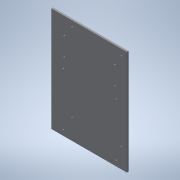
# Autodesk Inventor part: Akrilik
Saved by Autodesk Inventor 2020 (Build 240168000, 168)
## iProperties
Created: 2021-04-23
Part Number: Akrilik
Material: Generic
Document SubType Name: Modeling
Designer: scrip
Density: 1 g/cm^3
Appearance: Default
Author: scrip
Autodesk Inventor part; units mm, degrees
ref_plane "YZ Plane" through (0, 0, 0) normal (1, 0, 0) x (0, 1, 0)
ref_plane "XZ Plane" through (0, 0, 0) normal (0, 1, 0) x (-1, 0, 0)
ref_plane "XY Plane" through (0, 0, 0) normal (0, 0, 1) x (1, 0, 0)
sketch "Sketch1" plane through (0, 0, 0) normal (0, 0, 1) x (1, 0, 0)
  line L0 (-43.437, -19.7437) -> (55.293, -19.7437)
  line L1 (55.293, -19.7437) -> (55.293, -118.7837)
  circle A0 centre (6.169, -65.1647) radius 0.508
  circle A1 centre (-0.333, -65.1647) radius 0.508
  arc A2 (23.1745, -85.9924) -> (23.1745, -82.9951) centre (23.238, -84.4937) ccw
  arc A3 (23.1745, -82.9951) -> (23.1745, -85.9924) centre (23.111, -84.4937) ccw
  circle A4 centre (-11.179, -100.7497) radius 0.75
  circle A5 centre (28.445, -83.4777) radius 0.75
  circle A6 centre (36.573, -92.1137) radius 0.508
  circle A7 centre (-30.737, -64.3737) radius 0.4
  circle A8 centre (-25.657, -64.3737) radius 0.4
  circle A9 centre (-33.277, -89.3737) radius 0.4
  circle A10 centre (-28.197, -89.3737) radius 0.4
  circle A11 centre (-23.117, -89.3737) radius 0.4
  circle A12 centre (-12.957, -41.3137) radius 0.508
  circle A13 centre (-7.877, -41.3137) radius 0.508
  circle A14 centre (-12.957, -32.4237) radius 0.508
  circle A15 centre (-7.877, -32.4237) radius 0.508
  circle A16 centre (-25.657, -98.4637) radius 0.508
  circle A17 centre (-30.737, -98.4637) radius 0.508
  circle A18 centre (-29.467, -32.4237) radius 0.508
  circle A19 centre (-24.387, -32.4237) radius 0.508
  circle A20 centre (-14.227, -60.3637) radius 0.55
  circle A21 centre (-32.007, -71.7937) radius 0.508
  circle A22 centre (-26.927, -71.7937) radius 0.508
  circle A23 centre (-21.847, -71.7937) radius 0.508
  circle A24 centre (-14.227, -71.7937) radius 0.508
  circle A25 centre (-9.147, -71.7937) radius 0.508
  circle A26 centre (-4.067, -71.7937) radius 0.508
  circle A27 centre (-32.007, -23.5337) radius 0.508
  circle A28 centre (-26.927, -23.5337) radius 0.508
  circle A29 centre (-21.847, -23.5337) radius 0.508
  circle A30 centre (-16.767, -23.5337) radius 0.508
  circle A31 centre (-10.163, -23.5337) radius 0.508
  circle A32 centre (-5.083, -23.5337) radius 0.508
  circle A33 centre (-0.003, -23.5337) radius 0.508
  circle A34 centre (5.077, -23.5337) radius 0.508
  circle A35 centre (-39.627, -23.5337) radius 1.5
  circle A36 centre (51.813, -114.9737) radius 1.5
  circle A37 centre (-37.087, -38.7737) radius 1.6
  circle A38 centre (-7.877, -51.4737) radius 0.55
  circle A39 centre (-9.147, -60.3637) radius 0.55
  circle A40 centre (-7.877, -46.3937) radius 0.55
  circle A41 centre (13.713, -23.5337) radius 1.6
  circle A42 centre (-37.087, -66.7137) radius 1.6
  circle A43 centre (-39.627, -114.9737) radius 1.5
  circle A44 centre (51.813, -23.5337) radius 1.5
  circle A45 centre (2.537, -23.5337) radius 0.508
  circle A46 centre (-2.543, -23.5337) radius 0.508
  circle A47 centre (-7.623, -23.5337) radius 0.508
  circle A48 centre (-12.703, -23.5337) radius 0.508
  circle A49 centre (-19.307, -23.5337) radius 0.508
  circle A50 centre (-24.387, -23.5337) radius 0.508
  circle A51 centre (-29.467, -23.5337) radius 0.508
  circle A52 centre (-34.547, -23.5337) radius 0.508
  circle A53 centre (-6.607, -71.7937) radius 0.508
  circle A54 centre (-11.687, -71.7937) radius 0.508
  circle A55 centre (-16.767, -71.7937) radius 0.508
  circle A56 centre (-24.387, -71.7937) radius 0.508
  circle A57 centre (-29.467, -71.7937) radius 0.508
  circle A58 centre (-34.547, -71.7937) radius 0.508
  circle A59 centre (-21.847, -32.4237) radius 0.508
  circle A60 centre (-26.927, -32.4237) radius 0.508
  circle A61 centre (-33.277, -98.4637) radius 0.508
  circle A62 centre (-28.197, -98.4637) radius 0.508
  circle A63 centre (-5.337, -32.4237) radius 0.508
  circle A64 centre (-10.417, -32.4237) radius 0.508
  circle A65 centre (-5.337, -41.3137) radius 0.508
  circle A66 centre (-10.417, -41.3137) radius 0.508
  circle A67 centre (-20.577, -89.3737) radius 0.4
  circle A68 centre (-25.657, -89.3737) radius 0.4
  circle A69 centre (-30.737, -89.3737) radius 0.4
  circle A70 centre (-23.117, -64.3737) radius 0.4
  circle A71 centre (-28.197, -64.3737) radius 0.4
  circle A72 centre (36.573, -89.5737) radius 0.508
  circle A73 centre (36.573, -94.6537) radius 0.508
  circle A74 centre (28.445, -100.7497) radius 0.75
  circle A75 centre (-11.179, -83.4777) radius 0.75
  circle A76 centre (-6.607, -99.7337) radius 1.5
  circle A77 centre (-0.333, -60.6427) radius 0.508
  circle A78 centre (6.169, -60.6427) radius 0.508
  line L2 (55.293, -118.7837) -> (-43.437, -118.7837)
  line L3 (55.293, -19.7437) -> (55.293, -118.7837)
  line L4 (-43.437, -19.7437) -> (55.293, -19.7437)
  line L5 (-43.437, -118.7837) -> (-43.437, -19.7437)
  line L6 (-59.627, 55.0712) -> (-59.627, -124.9737)
  line L7 (-59.627, -124.9737) -> (70.373, -124.9737)
  line L8 (70.373, -124.9737) -> (70.373, 55.0712)
  line L9 (70.373, 55.0712) -> (-59.627, 55.0712)
  arc A79 (-37.9994, -7.7176) -> (-37.9994, -3.2176) centre (-37.9994, -5.4676) ccw
  arc A80 (-37.9994, 23.973) -> (-37.9994, 28.473) centre (-37.9994, 26.223) ccw
  arc A81 (49.0006, -3.2176) -> (49.0006, -7.7176) centre (49.0006, -5.4676) ccw
  arc A82 (49.0006, 28.473) -> (49.0006, 23.973) centre (49.0006, 26.223) ccw
  circle A83 centre (-39.627, -23.5337) radius 1.5
  circle A84 centre (-39.627, -114.9737) radius 1.5
  circle A85 centre (51.813, -114.9737) radius 1.5
  circle A86 centre (51.813, -23.5337) radius 1.5
  circle A87 centre (49.0006, -5.4676) radius 1.5
  circle A88 centre (49.0006, 26.223) radius 1.5
  circle A89 centre (-37.9994, 26.223) radius 1.1903
  circle A90 centre (-37.9994, -5.4676) radius 1.5
  point P0 (0, 0)
  point P1 (-30.337, -14.7437)
  point P2 (19.4617, -123.7837)
  point P3 (60.293, -53.7773)
  point P4 (-48.437, -58.5398)
extrude "Extrusion1" add sketch "Sketch1" along normal blind 3 contours L0 L1 L2 L5 | A0 | A1 | A3 A2 | A4 | A5 | A6 | A7 | A8 | A9 | A10 | A11 | A12 | A13 | A14 | A15 | A16 | A17 | A18 | A19 | A20 | A21 | A22 | A23 | A24 | A25 | A26 | A27 | A28 | A29 | A30 | A31 | A32 | A33 | A34 | A35 | A36 | A37 | A38 | A39 | A40 | A41 | A42 | A43 | A44 | A45 | A46 | A47 | A48 | A49 | A50 | A51 | A52 | A53 | A54 | A55 | A56 | A57 | A58 | A59 | A60 | A61 | A62 | A63 | A64 | A65 | A66 | A67 | A68 | A69 | A70 | A71 | A72 | A73 | A74 | A75 | A76 | A77 | A78 | L9 L8 L7 L6 | A87 | A88 | A89 | A90
sketch "Sketch6" plane through (0, 0, 0) normal (0, 0, -1) x (-1, 0, 0)
  arc A0 (37.9994, 28.473) -> (37.9994, 23.973) centre (37.9994, 26.223) ccw projected
  arc A1 (37.9994, -3.2176) -> (37.9994, -7.7176) centre (37.9994, -5.4676) ccw projected
  arc A2 (-49.0006, 23.973) -> (-49.0006, 28.473) centre (-49.0006, 26.223) ccw projected
  arc A3 (-49.0006, -7.7176) -> (-49.0006, -3.2176) centre (-49.0006, -5.4676) ccw projected
  arc A4 (-49.0006, 23.973) -> (-49.0006, 28.473) centre (-49.0006, 26.223) ccw projected
  arc A5 (-49.0006, 23.973) -> (-49.0006, 28.473) centre (-49.0006, 26.223) ccw projected
  arc A6 (-49.0006, 23.973) -> (-49.0006, 28.473) centre (-49.0006, 26.223) ccw projected
  point P0 (0, 0)
sketch "Sketch7" plane through (0, 0, 3) normal (0, 0, 1) x (1, 0, 0)
  arc A0 (49.0006, 28.473) -> (49.0006, 23.973) centre (49.0006, 26.223) ccw projected
  arc A1 (49.0006, -3.2176) -> (49.0006, -7.7176) centre (49.0006, -5.4676) ccw projected
  arc A2 (-37.9994, -7.7176) -> (-37.9994, -3.2176) centre (-37.9994, -5.4676) ccw projected
  arc A3 (-37.9994, 23.973) -> (-37.9994, 28.473) centre (-37.9994, 26.223) ccw projected
  circle A4 centre (-39.627, -114.9737) radius 1.5 projected
  circle A5 centre (-39.627, -23.5337) radius 1.5 projected
  circle A6 centre (51.813, -23.5337) radius 1.5 projected
  circle A7 centre (51.813, -114.9737) radius 1.5 projected
  point P0 (0, 0)
hole "Hole5" at (49.0006, 26.223, 3) at (49.0006, -5.4676, 3) at (-37.9994, 26.223, 3) at (-37.9994, -5.4676, 3) at (-39.627, -23.5337, 3) at (51.813, -23.5337, 3) at (51.813, -114.9737, 3) at (-39.627, -114.9737, 3) direction (0, 0, -1) diameter 3 end through all
sketch "Sketch8" plane through (0, 0, 3) normal (0, 0, 1) x (1, 0, 0)
  line L0 (70.373, 55.0712) -> (-59.627, 55.0712) projected
  line L1 (70.373, -124.9737) -> (70.373, 55.0712) projected
  point P0 (0, 0)
  point P1 (60.373, 45.0712)
  point P2 (-24.627, 46.0375)
  point P3 (60.373, -89.9288)
  point P4 (-24.627, -88.9625)
  dimension "d61" = 10
  dimension "d62" = 10
  dimension "d63" = 85
  dimension "d64" = 135
  dimension "d65" = 135
  measures "d61" distance from line of L0 point (60.373, 45.071)
  measures "d62" distance from line of L1 point (60.373, 45.071)
  measures "d63" horizontal distance of point (-24.627, 46.038) point (60.373, 45.071)
  measures "d64" distance of point (60.373, -89.929) point (60.373, 45.071)
  measures "d65" distance of point (-24.627, 46.038) point (-24.627, -88.962)
hole "Hole6" at (60.373, 45.0712, 3) at (60.373, -89.9288, 3) at (-24.627, -88.9625, 3) at (-24.627, 46.0375, 3) direction (0, 0, -1) diameter 3 end through all
body "Solid1"
